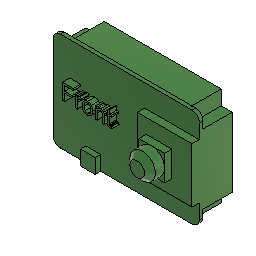
ESP32-CAM-Case (Autodesk Fusion 360 archive; units mm, degrees)
design "AI-Thinker-ESP32-CAM"
Autodesk Fusion 360 part; units mm, degrees
sketch "Sketch1" plane through (0, 0, 0) normal (0, 1, 0) x (1, 0, 0)
  line L0 (0, 0) -> (40, 0)
  line L1 (40, 0) -> (40, -27)
  line L2 (40, -27) -> (0, -27)
  line L3 (0, -27) -> (0, 0)
  circle A0 centre (2, -25) radius 2
  circle A1 centre (2, -2) radius 2
  circle A2 centre (38, -25) radius 2
  circle A3 centre (38, -2) radius 2
  dimension "d1" = 40
  dimension "d2" = 27
  dimension "d3" = 4
  dimension "d4" = 4
  dimension "d5" = 4
  constraint horizontal L0
  constraint vertical L1
  constraint horizontal L2
  constraint vertical L3
  constraint coincident L0.start L3.end
  constraint tangent L2 A0
  measures "d1" distance of L0.start L0.end
  measures "d2" distance of L0.start L2.end
  measures "d3" diameter of A1
  measures "d4" diameter of A2
  measures "d5" diameter of A3
extrude "Extrude1" add sketch "Sketch1" along normal blind 1 contours L0 L1 L2 L3 A0 A1 A2 A3 | A1 | A3 | A0 | A2
sketch "Sketch2" plane through (0, 0, 0) normal (0, -1, 0) x (1, 0, 0)
  arc A0 (40, 25.0009) -> (38.0007, 27) centre (38, 25) ccw
  line L0 (38.0007, 27) -> (2, 27)
  arc A1 (2, 27) -> (0, 25) centre (2, 25) ccw
  line L1 (0, 25) -> (0, 2)
  arc A2 (0, 2) -> (2, 0) centre (2, 2) ccw
  line L2 (2, 0) -> (38, 0)
  arc A3 (38, 0) -> (40, 2.0009) centre (38, 2) ccw
  line L3 (40, 2.0009) -> (40, 25.0009)
  line L4 (40.0642, 27) -> (25.0642, 27)
  line L5 (25.0642, 27) -> (25.0642, 13.5)
  line L6 (25.0642, 13.5) -> (40.0642, 13.5)
  line L7 (40.0642, 13.5) -> (40.0642, 27)
  line L8 (25.0642, 13.5) -> (40.0642, 13.5)
  line L9 (40.0642, 13.5) -> (40.0642, 6)
  line L10 (40.0642, 6) -> (25.0642, 6)
  line L11 (25.0642, 6) -> (25.0642, 13.5)
  line L12 (25.0642, 13.5) -> (40.0642, 13.5)
  line L13 (40.0642, 13.5) -> (40.0642, 21)
  line L14 (40.0642, 21) -> (25.0642, 21)
  line L15 (25.0642, 21) -> (25.0642, 13.5)
  dimension "d8" = 15
  dimension "d9" = 13.5
  dimension "d10" = 7.5
  dimension "d11" = 7.5
  constraint horizontal L4
  constraint vertical L5
  constraint horizontal L6
  constraint vertical L7
  constraint horizontal L8
  constraint vertical L9
  constraint horizontal L10
  constraint vertical L11
  constraint horizontal L12
  constraint vertical L13
  constraint horizontal L14
  constraint vertical L15
  measures "d8" distance of L4.start L4.end
  measures "d9" distance of L4.start L6.end
  measures "d10" distance of L5.end L10.end
  measures "d11" distance of L5.end L14.end
extrude "Extrude2" add sketch "Sketch2" along normal blind 2 contours L3 L5 L6 L8 L12 L14 L15 | L3 L6 L8 L10 L11 L12
sketch "Sketch3" plane through (0, -2, 0) normal (0, -1, 0) x (1, 0, 0)
  line L0 (40, 6) -> (40, 21)
  line L1 (40, 21) -> (25.0642, 21)
  line L2 (25.0642, 21) -> (25.0642, 6)
  line L3 (25.0642, 6) -> (40, 6)
  line L4 (40, 21) -> (31, 21)
  line L5 (31, 21) -> (31, 13.5)
  line L6 (31, 13.5) -> (34.5, 13.5)
  line L7 (34.5, 13.5) -> (34.5, 10)
  line L8 (34.5, 10) -> (27.5, 10)
  line L9 (27.5, 10) -> (27.5, 17)
  line L10 (27.5, 17) -> (34.5, 17)
  line L11 (34.5, 17) -> (34.5, 10)
  dimension "d14" = 9
  dimension "d15" = 3.5
  dimension "d16" = 3.5
  dimension "d17" = 7
  dimension "d18" = 7
  constraint coincident L0.end L1.start
  constraint perpendicular L0 L4
  constraint perpendicular L4 L5
  constraint perpendicular L0 L6
  constraint perpendicular L6 L7
  constraint horizontal L8
  constraint vertical L9
  constraint horizontal L10
  constraint vertical L11
  measures "d14" distance of L0.end L4.end
  measures "d15" distance of L5.end L6.end
  measures "d16" distance of L6.end L7.end
  measures "d17" distance of L7.end L10.end
  measures "d18" distance of L7.end L8.end
extrude "Extrude3" add sketch "Sketch3" along normal blind 2 contours L5 L6 L10 L11 | L5 L6 L7 L8 L9 L10 L11
sketch "Sketch4" plane through (0, -4, 0) normal (0, -1, 0) x (1, 0, 0)
  line L0 (34.5, 17) -> (27.5, 17)
  line L1 (27.5, 17) -> (27.5, 10)
  line L2 (27.5, 10) -> (34.5, 10)
  line L3 (34.5, 10) -> (34.5, 17)
  line L4 (27.5, 17) -> (34.5, 10)
  line L5 (34.5, 17) -> (27.5, 10)
  circle A0 centre (31, 13.5) radius 3.5
  constraint coincident L0.end L1.start
  constraint coincident L2.end L3.start
  constraint coincident L0.start L3.end
  constraint coincident L1.end L2.start
  constraint midpoint L4 A0.centre
  constraint tangent L3 A0
extrude "Extrude4" add sketch "Sketch4" along normal blind 4 contours L4 L5 A0 | L4 L5 A0 | L4 L5 A0 | L4 L5 A0
chamfer "Chamfer1" distance 1.5 angle 45 1 edges at (27.7369, -8, 12.2343)
sketch "Sketch5" plane through (0, 0, 0) normal (0, -1, 0) x (1, 0, 0)
  line L0 (25.0642, 21) -> (40, 21)
  line L1 (40, 21) -> (40, 25.0009)
  arc A0 (40, 25.0009) -> (38.0007, 27) centre (38, 25) ccw
  line L2 (38.0007, 27) -> (2, 27)
  arc A1 (2, 27) -> (0, 25) centre (2, 25) ccw
  line L3 (0, 25) -> (0, 2)
  arc A2 (0, 2) -> (2, 0) centre (2, 2) ccw
  line L4 (2, 0) -> (38, 0)
  arc A3 (38, 0) -> (40, 2.0009) centre (38, 2) ccw
  line L5 (40, 2.0009) -> (40, 6)
  line L6 (40, 6) -> (25.0642, 6)
  line L7 (25.0642, 6) -> (25.0642, 21)
  line L8 (0, 0) -> (13, 0)
  line L9 (13, 0) -> (13, 4)
  line L10 (13, 4) -> (0, 4)
  line L11 (0, 4) -> (0, 0)
  line L12 (13, 4) -> (9, 4)
  line L13 (9, 4) -> (9, 0)
  line L14 (9, 0) -> (13, 0)
  line L15 (13, 0) -> (13, 4)
  dimension "d24" = 13
  dimension "d25" = 4
  dimension "d26" = 4
  constraint horizontal L8
  constraint vertical L9
  constraint horizontal L10
  constraint vertical L11
  constraint coincident L8.start L11.end
  constraint horizontal L12
  constraint vertical L13
  constraint horizontal L14
  constraint vertical L15
  measures "d24" distance of L8.start L8.end
  measures "d25" distance of L8.start L10.end
  measures "d26" distance of L9.end L12.end
extrude "Extrude5" add sketch "Sketch5" along normal blind 1.5 contours L4 L8 L9 L10 L12 L13 L14 L15
sketch "Sketch6" plane through (0, 1, 0) normal (0, 1, 0) x (-1, 0, 0)
  arc A0 (-38.0007, 27) -> (-40, 25.0009) centre (-38, 25) ccw
  line L0 (-40, 25.0009) -> (-40, 2.0009)
  arc A1 (-40, 2.0009) -> (-38, 0) centre (-38, 2) ccw
  line L1 (-38, 0) -> (-2, 0)
  arc A2 (-2, 0) -> (0, 2) centre (-2, 2) ccw
  line L2 (0, 2) -> (0, 25)
  arc A3 (0, 25) -> (-2, 27) centre (-2, 25) ccw
  line L3 (-2, 27) -> (-38.0007, 27)
  line L4 (-40, 0) -> (-37, 0)
  line L5 (-37, 0) -> (-37, 4)
  line L6 (-37, 4) -> (-40, 4)
  line L7 (-40, 4) -> (-40, 0)
  line L8 (-37, 4) -> (-40, 4)
  line L9 (-40, 4) -> (-40, 27)
  line L10 (-40, 27) -> (-37, 27)
  line L11 (-37, 27) -> (-37, 4)
  line L12 (-37, 27) -> (-40, 27)
  line L13 (-40, 27) -> (-40, 23)
  line L14 (-40, 23) -> (-37, 23)
  line L15 (-37, 23) -> (-37, 27)
  line L16 (0, 0) -> (-5, 0)
  line L17 (-5, 0) -> (-5, 4)
  line L18 (-5, 4) -> (0, 4)
  line L19 (0, 4) -> (0, 0)
  line L20 (-5, 4) -> (0, 4)
  line L21 (0, 4) -> (0, 27)
  line L22 (0, 27) -> (-5, 27)
  line L23 (-5, 27) -> (-5, 4)
  line L24 (-5, 27) -> (0, 27)
  line L25 (0, 27) -> (0, 23)
  line L26 (0, 23) -> (-5, 23)
  line L27 (-5, 23) -> (-5, 27)
  dimension "d29" = 3
  dimension "d30" = 4
  dimension "d31" = 5
  dimension "d32" = 4
  dimension "d33" = 4
  constraint horizontal L4
  constraint vertical L5
  constraint horizontal L6
  constraint vertical L7
  constraint horizontal L8
  constraint vertical L9
  constraint horizontal L10
  constraint vertical L11
  constraint horizontal L12
  constraint vertical L13
  constraint horizontal L14
  constraint vertical L15
  constraint coincident L9 L13.end
  constraint horizontal L16
  constraint vertical L17
  constraint horizontal L18
  constraint vertical L19
  constraint coincident L16.start L19.end
  constraint horizontal L20
  constraint vertical L21
  constraint horizontal L22
  constraint vertical L23
  constraint horizontal L24
  constraint vertical L25
  constraint horizontal L26
  constraint vertical L27
  measures "d29" distance of L4.start L4.end
  measures "d30" distance of L4.start L6.end
  measures "d31" distance of L16.start L16.end
  measures "d32" distance of L16.start L18.end
  measures "d33" distance of L22.end L26.end
extrude "Extrude6" add sketch "Sketch6" along normal blind 8 contours L1 L3 L5 L11 L15 L17 L23 L27 | L0 L6 L8 L9 L11 L14 | L2 L18 L20 L21 L23 L26
sketch "Sketch7" plane through (0, 0, 0) normal (0, -1, 0) x (1, 0, 0)
  line L0 (9, 0) -> (9, 4)
  line L1 (9, 4) -> (13, 4)
  line L2 (13, 4) -> (13, 0)
  line L3 (13, 0) -> (38, 0)
  arc A0 (38, 0) -> (40, 2.0009) centre (38, 2) ccw
  line L4 (40, 2.0009) -> (40, 6)
  line L5 (40, 6) -> (25.0642, 6)
  line L6 (25.0642, 6) -> (25.0642, 21)
  line L7 (25.0642, 21) -> (40, 21)
  line L8 (40, 21) -> (40, 25.0009)
  arc A1 (40, 25.0009) -> (38.0007, 27) centre (38, 25) ccw
  line L9 (38.0007, 27) -> (2, 27)
  arc A2 (2, 27) -> (0, 25) centre (2, 25) ccw
  line L10 (0, 25) -> (0, 2)
  arc A3 (0, 2) -> (2, 0) centre (2, 2) ccw
  line L11 (2, 0) -> (9, 0)
  line L12 (4.5973, 13.5903) -> (4.5973, 17.8852)
  line L13 (4.5973, 17.8852) -> (7.4948, 17.8852)
  line L14 (7.4948, 17.8852) -> (7.4948, 17.3784)
  line L15 (7.4948, 17.3784) -> (5.1657, 17.3784)
  line L16 (5.1657, 17.3784) -> (5.1657, 16.0483)
  line L17 (5.1657, 16.0483) -> (7.1813, 16.0483)
  line L18 (7.1813, 16.0483) -> (7.1813, 15.5415)
  line L19 (7.1813, 15.5415) -> (5.1657, 15.5415)
  line L20 (5.1657, 15.5415) -> (5.1657, 13.5903)
  line L21 (5.1657, 13.5903) -> (4.5973, 13.5903)
  line L22 (8.1598, 13.5903) -> (8.1598, 16.7016)
  line L23 (8.1598, 16.7016) -> (8.6344, 16.7016)
  line L24 (8.6344, 16.7016) -> (8.6344, 16.23)
  spline S0 degree 3 poles (8.6344, 16.23) (8.6873, 16.3258) (8.7772, 16.4888) (8.9136, 16.6146) (8.9699, 16.6665) knots 0 0 0 0 0.03255 0.055364 0.055364 0.055364 0.055364
  spline S1 degree 3 poles (8.9699, 16.6665) (9.0223, 16.6972) (9.127, 16.7586) (9.2479, 16.7675) (9.3082, 16.772) knots 0 0 0 0 0.017983 0.035867 0.035867 0.035867 0.035867
  spline S2 degree 3 poles (9.3082, 16.772) (9.3996, 16.7635) (9.5921, 16.7458) (9.7613, 16.6516) (9.8502, 16.602) knots 0 0 0 0 0.027214 0.057359 0.057359 0.057359 0.057359
  line L25 (9.8502, 16.602) -> (9.6686, 16.1128)
  spline S3 degree 3 poles (9.6686, 16.1128) (9.6055, 16.1461) (9.4841, 16.2102) (9.3475, 16.2216) (9.2819, 16.227) knots 0 0 0 0 0.02115 0.040696 0.040696 0.040696 0.040696
  spline S4 degree 3 poles (9.2819, 16.227) (9.2257, 16.2227) (9.1135, 16.2141) (9.0187, 16.1534) (8.9713, 16.123) knots 0 0 0 0 0.016611 0.033207 0.033207 0.033207 0.033207
  spline S5 degree 3 poles (8.9713, 16.123) (8.9284, 16.0841) (8.8399, 16.0038) (8.7971, 15.892) (8.775, 15.8345) knots 0 0 0 0 0.017122 0.035337 0.035337 0.035337 0.035337
  spline S6 degree 3 poles (8.775, 15.8345) (8.7494, 15.7368) (8.6965, 15.5352) (8.6903, 15.3268) (8.6871, 15.2192) knots 0 0 0 0 0.030172 0.062327 0.062327 0.062327 0.062327
  line L26 (8.6871, 15.2192) -> (8.6871, 13.5903)
  line L27 (8.6871, 13.5903) -> (8.1598, 13.5903)
  spline S7 degree 3 poles (9.9674, 15.146) (9.9794, 15.4079) (10.0015, 15.8895) (10.308, 16.2581) (10.4479, 16.4263) knots 0 0 0 0 0.076173 0.140104 0.140104 0.140104 0.140104
  spline S8 degree 3 poles (10.4479, 16.4263) (10.5912, 16.5271) (10.8846, 16.7336) (11.243, 16.759) (11.4264, 16.772) knots 0 0 0 0 0.051529 0.105546 0.105546 0.105546 0.105546
  spline S9 degree 3 poles (11.4264, 16.772) (11.6286, 16.7563) (12.0229, 16.7259) (12.3271, 16.4741) (12.4752, 16.3515) knots 0 0 0 0 0.059241 0.115491 0.115491 0.115491 0.115491
  spline S10 degree 3 poles (12.4752, 16.3515) (12.5939, 16.1908) (12.8478, 15.8468) (12.8704, 15.4183) (12.8825, 15.1899) knots 0 0 0 0 0.058642 0.125523 0.125523 0.125523 0.125523
  spline S11 degree 3 poles (12.8825, 15.1899) (12.8789, 15.0087) (12.8726, 14.6828) (12.7547, 14.3797) (12.7023, 14.2451) knots 0 0 0 0 0.053839 0.096849 0.096849 0.096849 0.096849
  spline S12 degree 3 poles (12.7023, 14.2451) (12.6352, 14.1367) (12.5006, 13.9191) (12.2857, 13.7801) (12.1779, 13.7104) knots 0 0 0 0 0.03774 0.075731 0.075731 0.075731 0.075731
  spline S13 degree 3 poles (12.1779, 13.7104) (12.0599, 13.6549) (11.8218, 13.5428) (11.559, 13.5276) (11.4264, 13.52) knots 0 0 0 0 0.038728 0.078165 0.078165 0.078165 0.078165
  spline S14 degree 3 poles (11.4264, 13.52) (11.2215, 13.535) (10.8247, 13.5641) (10.5183, 13.8168) (10.3702, 13.9389) knots 0 0 0 0 0.059991 0.116149 0.116149 0.116149 0.116149
  spline S15 degree 3 poles (10.3702, 13.9389) (10.253, 14.1035) (9.9969, 14.4629) (9.9778, 14.9059) (9.9674, 15.146) knots 0 0 0 0 0.059383 0.129688 0.129688 0.129688 0.129688
  spline S16 degree 3 poles (10.5094, 15.146) (10.5145, 14.9666) (10.5236, 14.6438) (10.6943, 14.3718) (10.7701, 14.251) knots 0 0 0 0 0.052663 0.094729 0.094729 0.094729 0.094729
  spline S17 degree 3 poles (10.7701, 14.251) (10.8627, 14.1642) (11.0477, 13.9908) (11.3002, 13.966) (11.4264, 13.9536) knots 0 0 0 0 0.036936 0.073874 0.073874 0.073874 0.073874
  spline S18 degree 3 poles (11.4264, 13.9536) (11.5519, 13.9662) (11.8036, 13.9915) (11.9875, 14.1653) (12.0797, 14.2524) knots 0 0 0 0 0.03673 0.073674 0.073674 0.073674 0.073674
  spline S19 degree 3 poles (12.0797, 14.2524) (12.1555, 14.3749) (12.3272, 14.6524) (12.3357, 14.9803) (12.3405, 15.1636) knots 0 0 0 0 0.042488 0.096278 0.096278 0.096278 0.096278
  spline S20 degree 3 poles (12.3405, 15.1636) (12.3348, 15.3378) (12.3244, 15.654) (12.1545, 15.9191) (12.0783, 16.0381) knots 0 0 0 0 0.051142 0.092806 0.092806 0.092806 0.092806
  spline S21 degree 3 poles (12.0783, 16.0381) (11.9859, 16.1248) (11.802, 16.2974) (11.5512, 16.3228) (11.4264, 16.3354) knots 0 0 0 0 0.036907 0.07345 0.07345 0.07345 0.07345
  spline S22 degree 3 poles (11.4264, 16.3354) (11.3002, 16.3231) (11.048, 16.2986) (10.8627, 16.1258) (10.7701, 16.0395) knots 0 0 0 0 0.03693 0.0738 0.0738 0.0738 0.0738
  spline S23 degree 3 poles (10.7701, 16.0395) (10.6943, 15.9191) (10.5235, 15.6476) (10.5144, 15.3253) (10.5094, 15.146) knots 0 0 0 0 0.041968 0.094595 0.094595 0.094595 0.094595
  line L28 (13.5006, 13.5903) -> (13.5006, 16.7016)
  line L29 (13.5006, 16.7016) -> (13.9752, 16.7016)
  line L30 (13.9752, 16.7016) -> (13.9752, 16.2593)
  spline S24 degree 3 poles (13.9752, 16.2593) (14.1037, 16.4088) (14.3645, 16.7123) (14.7632, 16.7519) (14.9655, 16.772) knots 0 0 0 0 0.056866 0.115415 0.115415 0.115415 0.115415
  spline S25 degree 3 poles (14.9655, 16.772) (15.0563, 16.7682) (15.2339, 16.7607) (15.401, 16.7004) (15.4825, 16.6709) knots 0 0 0 0 0.027108 0.052963 0.052963 0.052963 0.052963
  spline S26 degree 3 poles (15.4825, 16.6709) (15.5548, 16.6365) (15.6906, 16.5719) (15.7893, 16.4587) (15.8356, 16.4057) knots 0 0 0 0 0.023697 0.044569 0.044569 0.044569 0.044569
  spline S27 degree 3 poles (15.8356, 16.4057) (15.872, 16.3473) (15.9473, 16.2262) (15.9818, 16.0877) (15.9996, 16.0161) knots 0 0 0 0 0.020524 0.04251 0.04251 0.04251 0.04251
  spline S28 degree 3 poles (15.9996, 16.0161) (16.0081, 15.949) (16.0295, 15.7789) (16.0292, 15.6073) (16.0289, 15.5034) knots 0 0 0 0 0.020261 0.051398 0.051398 0.051398 0.051398
  line L31 (16.0289, 15.5034) -> (16.0289, 13.5903)
  line L32 (16.0289, 13.5903) -> (15.5016, 13.5903)
  line L33 (15.5016, 13.5903) -> (15.5016, 15.4829)
  spline S29 degree 3 poles (15.5016, 15.4829) (15.5011, 15.5774) (15.5002, 15.7408) (15.4579, 15.8984) (15.4401, 15.9648) knots 0 0 0 0 0.028204 0.04876 0.04876 0.04876 0.04876
  spline S30 degree 3 poles (15.4401, 15.9648) (15.4151, 16.0156) (15.3643, 16.1192) (15.2699, 16.1858) (15.2218, 16.2197) knots 0 0 0 0 0.0167 0.034039 0.034039 0.034039 0.034039
  spline S31 degree 3 poles (15.2218, 16.2197) (15.1661, 16.2475) (15.0504, 16.3051) (14.9211, 16.3116) (14.8541, 16.3149) knots 0 0 0 0 0.018466 0.038347 0.038347 0.038347 0.038347
  spline S32 degree 3 poles (14.8541, 16.3149) (14.7461, 16.3064) (14.5321, 16.2894) (14.3585, 16.1634) (14.2726, 16.1011) knots 0 0 0 0 0.031837 0.063044 0.063044 0.063044 0.063044
  spline S33 degree 3 poles (14.2726, 16.1011) (14.2017, 16.0011) (14.0314, 15.7608) (14.0292, 15.4633) (14.028, 15.2895) knots 0 0 0 0 0.036006 0.086549 0.086549 0.086549 0.086549
  line L34 (14.028, 15.2895) -> (14.028, 13.5903)
  line L35 (14.028, 13.5903) -> (13.5006, 13.5903)
  line L36 (17.9889, 14.062) -> (18.0651, 13.5962)
  spline S34 degree 3 poles (18.0651, 13.5962) (17.995, 13.5825) (17.8633, 13.5569) (17.7293, 13.5517) (17.6666, 13.5493) knots 0 0 0 0 0.021385 0.040171 0.040171 0.040171 0.040171
  spline S35 degree 3 poles (17.6666, 13.5493) (17.5804, 13.551) (17.4259, 13.5539) (17.284, 13.6137) (17.2213, 13.6401) knots 0 0 0 0 0.025589 0.045814 0.045814 0.045814 0.045814
  spline S36 degree 3 poles (17.2213, 13.6401) (17.1729, 13.6719) (17.0791, 13.7335) (17.0249, 13.8315) (16.9987, 13.8789) knots 0 0 0 0 0.01709 0.033088 0.033088 0.033088 0.033088
  spline S37 degree 3 poles (16.9987, 13.8789) (16.9801, 13.9551) (16.9306, 14.1591) (16.9328, 14.3696) (16.9342, 14.5014) knots 0 0 0 0 0.023465 0.062792 0.062792 0.062792 0.062792
  line L37 (16.9342, 14.5014) -> (16.9342, 16.2915)
  line L38 (16.9342, 16.2915) -> (16.5475, 16.2915)
  line L39 (16.5475, 16.2915) -> (16.5475, 16.7016)
  line L40 (16.5475, 16.7016) -> (16.9342, 16.7016)
  line L41 (16.9342, 16.7016) -> (16.9342, 17.4721)
  line L42 (16.9342, 17.4721) -> (17.4586, 17.7886)
  line L43 (17.4586, 17.7886) -> (17.4586, 16.7016)
  line L44 (17.4586, 16.7016) -> (17.9889, 16.7016)
  line L45 (17.9889, 16.7016) -> (17.9889, 16.2915)
  line L46 (17.9889, 16.2915) -> (17.4586, 16.2915)
  line L47 (17.4586, 16.2915) -> (17.4586, 14.4721)
  spline S38 degree 3 poles (17.4586, 14.4721) (17.4578, 14.41) (17.4566, 14.3121) (17.4785, 14.2169) (17.4865, 14.1821) knots 0 0 0 0 0.018543 0.029223 0.029223 0.029223 0.029223
  spline S39 degree 3 poles (17.4865, 14.1821) (17.4973, 14.1616) (17.5194, 14.1202) (17.5578, 14.0932) (17.5773, 14.0796) knots 0 0 0 0 0.006848 0.013872 0.013872 0.013872 0.013872
  spline S40 degree 3 poles (17.5773, 14.0796) (17.6024, 14.0685) (17.6596, 14.0433) (17.7223, 14.0421) (17.7575, 14.0415) knots 0 0 0 0 0.008169 0.018577 0.018577 0.018577 0.018577
  spline S41 degree 3 poles (17.7575, 14.0415) (17.7914, 14.0427) (17.8689, 14.0454) (17.9458, 14.056) (17.9889, 14.062) knots 0 0 0 0 0.010194 0.023248 0.023248 0.023248 0.023248
extrude "Extrude7" add sketch "Sketch7" along normal blind 2 contours L12 L13 L14 L15 L16 L17 L18 L19 L20 L21 | L22 L23 L24 S0 S1 S2 L25 S3 S4 S5 S6 L26 L27 | S7 S8 S9 S10 S11 S12 S13 S14 S15 | L28 L29 L30 S24 S25 S26 S27 S28 L31 L32 L33 S29 S30 S31 S32 S33 L34 L35 | L36 S34 S35 S36 S37 L37 L38 L39 L40 L41 L42 L43 L44 L45 L46 L47 S38 S39 S40 S41
